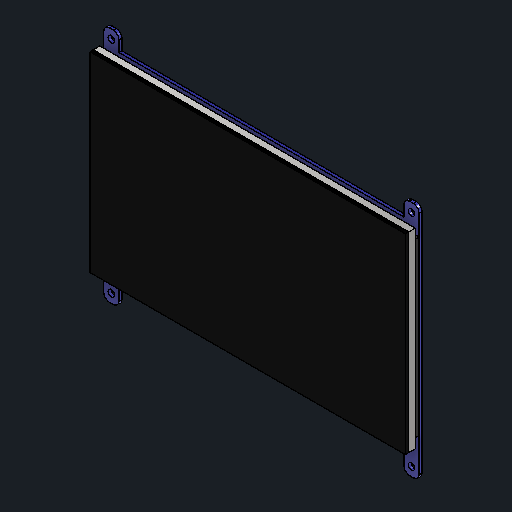
# Autodesk Inventor part: 7in Touch Display
Saved by Autodesk Inventor 2026.2 (Build 302298000, 298)
## iProperties
Created: 2026-01-20
Part Number: 7in Touch Display
Material: Generic
Document SubType Name: Modeling
Designer: JoshuaEah
Density: 1 g/cm^3
Appearance: Default
Author: JoshuaEah
Autodesk Inventor part; units mm, degrees
ref_plane "YZ Plane" through (0, 0, 0) normal (1, 0, 0) x (0, 1, 0)
ref_plane "XZ Plane" through (0, 0, 0) normal (0, 1, 0) x (-1, 0, 0)
ref_plane "XY Plane" through (0, 0, 0) normal (0, 0, 1) x (1, 0, 0)
sketch "Sketch1" plane through (0, 0, 0) normal (0, 0, 1) x (1, 0, 0)
  line L0 (0, 0) -> (164.9, 0)
  line L1 (164.9, 0) -> (164.9, 124.26)
  line L2 (164.9, 124.26) -> (0, 124.26)
  line L3 (0, 124.26) -> (0, 0)
  line L4 (8, 124.26) -> (8, 0)
  line L5 (8, 115.59) -> (156.9, 115.59)
  line L6 (82.45, 124.26) -> (82.45, 0)
  line L7 (0, 62.13) -> (164.9, 62.13)
  line L8 (156.9, 124.26) -> (156.9, 0)
  line L9 (8, 8.67) -> (156.9, 8.67)
  line L10 (4, 119.61) -> (4, 4.65) construction
  line L11 (4, 119.61) -> (160.9, 119.61) construction
  line L12 (160.9, 119.61) -> (160.9, 4.65) construction
  line L13 (4, 4.65) -> (160.9, 4.65) construction
  circle A0 centre (4, 119.61) radius 1.7
  circle A1 centre (160.9, 119.61) radius 1.7
  circle A2 centre (160.9, 4.65) radius 1.7
  circle A3 centre (4, 4.65) radius 1.7
  point P0 (156.9, 0)
  dimension "d0" = 164.9
  dimension "d1" = 124.26
  dimension "d18" = 106.92
  dimension "d21" = 156.9
  dimension "d22" = 114.96
  dimension "d23" = 3.4
  dimension "d24" = 148.9
  constraints: 28 end point, 8 symmetric about line, 4 centre point, 4 coincident, 4 midpoint, 4 point on line, 3 equal radius, 3 parallel, 2 perpendicular, 1 horizontal, 1 vertical
  measures "d0" distance of L2.end L1.end
  measures "d1" distance of L1.end L0.end
  measures "d18" diameter of L5 L7
  measures "d21" diameter of L10 L6
  measures "d22" diameter of L11 L7
  measures "d23" diameter of A0
  measures "d24" diameter of L4 L6
extrude "Extrusion1" add sketch "Sketch1" against normal blind 1.56 contours L3 L7 L4 L0 | L3 L2 L4 L7 | L4 L7 L6 L9 | L4 L5 L6 L7 | L8 L7 L1 L0 | L6 L7 L8 L9 | L6 L5 L8 L7 | L8 L2 L1 L7 | A0 | A1 | A2 | A3
fillet "Fillet1" radius 3 8 edges at (0, 124.26, -0.78) (8, 124.26, -0.78) (156.9, 124.26, -0.78) (164.9, 124.26, -0.78) (0, 0, -0.78) (8, 0, -0.78) (156.9, 0, -0.78) (164.9, 0, -0.78)
hole "Hole1" at (4, 119.61, 0) at (160.9, 119.61, 0) at (160.9, 4.65, 0) at (4, 4.65, 0) direction (0, 0, -1) diameter 3.4 end through all start extended yes clearance for "Flat Head Machine Screw" size "M3" standard "Ansi Metric M Profile"
sketch "Sketch3" plane through (0, 0, 0) normal (0, 0, 1) x (1, 0, 0)
  line L0 (0, 115.59) -> (164.9, 115.59)
  line L1 (164.9, 115.59) -> (164.9, 15.67)
  line L2 (164.9, 15.67) -> (0, 15.67)
  line L3 (0, 15.67) -> (0, 115.59)
  line L4 (0, 121.26) -> (0, 3) construction
  line L5 (164.9, 3) -> (164.9, 121.26) projected
  line L6 (8, 8.67) -> (156.9, 8.67) construction
  line L7 (156.9, 115.59) -> (8, 115.59) construction
  line L8 (15, 115.59) -> (15, 15.67)
  line L9 (82.45, 115.59) -> (82.45, 15.67)
  line L10 (149.9, 115.59) -> (149.9, 15.67)
  line L11 (0, 110.59) -> (164.9, 110.59)
  line L12 (164.9, 62.13) -> (0, 62.13)
  line L13 (0, 20.59) -> (164.9, 20.59)
  point P0 (15, 110.59)
  point P1 (15, 20.59)
  point P2 (149.9, 110.59)
  point P3 (149.9, 20.59)
  dimension "d35" = 7
  dimension "d38" = 15
  dimension "d43" = 5
  dimension "d44" = 90
  constraints: 20 end point, 9 point on line, 4 midpoint, 4 perpendicular, 2 parallel, 2 symmetric about line, 1 horizontal
  measures "d35" distance between parallel lines of L6 L2
  measures "d38" distance between parallel lines of L8 L3
  measures "d43" distance between parallel lines of L0 L11
  measures "d44" distance between parallel lines of L11 L13
extrude "Extrusion2" add sketch "Sketch3" along normal blind 2.04 separate body contours L11 L8 L12 L3 | L12 L8 L13 L3 | L11 L1 L12 L10 | L12 L1 L13 L10
extrude "Extrusion3" add sketch "Sketch3" along normal blind 3.45 from surface at 2.04 separate body
extrude "Extrusion4" add sketch "Sketch3" along normal blind 1.75 from surface at 5.49 separate body
